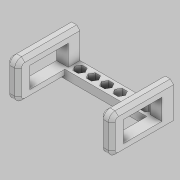
# Autodesk Inventor part: Chassis_atras_V4
Saved by Autodesk Inventor 2022.2 (Build 262287010, 287A)
## iProperties
Created: 2022-06-14
Part Number: Chassis_atras_V4
Material: Genérico
Document SubType Name: Modeling
Designer: Usuario
Density: 1 g/cm^3
Appearance: Valor por defecto
Author: Usuario
Autodesk Inventor part; units mm, degrees
ref_plane "YZ Plane" through (0, 0, 0) normal (1, 0, 0) x (0, 1, 0)
ref_plane "XZ Plane" through (0, 0, 0) normal (0, 1, 0) x (-1, 0, 0)
ref_plane "XY Plane" through (0, 0, 0) normal (0, 0, 1) x (1, 0, 0)
sketch "Boceto1" plane through (0, 0, 0) normal (0, 1, 0) x (-1, 0, 0)
  line L0 (29.505, -15) -> (44.5466, 0) construction
  line L1 (33.6552, -19.1617) -> (29.505, -15) construction
  line L2 (0, 0) -> (0, 6.3504) construction
  line L3 (0, 0) -> (0, -23.2363) construction
  line L4 (0, -14.2363) -> (24.5, -14.2363)
  line L5 (31.5, -23.2363) -> (31.5, 13.7637)
  line L6 (31.5, 13.7637) -> (24.5, 13.7637)
  line L7 (24.5, 13.7637) -> (24.5, -14.2363)
  line L8 (31.5, -23.2363) -> (0, -23.2363)
  line L9 (0, -14.2363) -> (-24.5, -14.2363)
  line L10 (-31.5, -23.2363) -> (-31.5, 13.7637)
  line L11 (-31.5, 13.7637) -> (-24.5, 13.7637)
  line L12 (-24.5, 13.7637) -> (-24.5, -14.2363)
  line L13 (-31.5, -23.2363) -> (0, -23.2363)
  dimension "d70" = 7
  dimension "d71" = 37
  dimension "d86" = 31.5
  dimension "d88" = 9
  constraints: 28 end point, 4 symmetric about line, 3 horizontal, 3 vertical, 1 perpendicular, 1 point on line
  measures "d70" distance of L5.end L6.end
  measures "d71" distance of L5.start L5.end
  measures "d86" distance of L3.end L5.start
  measures "d88" distance between parallel lines of L4 L8
extrude "Extrusión1" add sketch "Boceto1" along normal blind 5
sketch "Boceto11" plane through (0, 5, 0) normal (0, 1, 0) x (1, 0, 0)
  line L0 (-31.5, -13.7637) -> (-24.5, -13.7637) projected
  line L1 (31.5, 23.2363) -> (-31.5, 23.2363) projected
  line L2 (-31.5, -13.7637) -> (-24.5, -13.7637)
  line L3 (-24.5, -13.7637) -> (-24.5, 23.2363)
  line L4 (-24.5, 23.2363) -> (-31.5, 23.2363)
  line L5 (-31.5, 23.2363) -> (-31.5, -13.7637)
  line L6 (0, 0) -> (0, -8.2135) construction
  line L7 (31.5, -13.7637) -> (24.5, -13.7637)
  line L8 (24.5, -13.7637) -> (24.5, 23.2363)
  line L9 (24.5, 23.2363) -> (31.5, 23.2363)
  line L10 (31.5, 23.2363) -> (31.5, -13.7637)
  point P0 (31.5, 23.2363)
  point P1 (24.5, 23.2363)
  constraints: 18 end point, 6 symmetric about line, 2 parallel, 1 horizontal, 1 perpendicular, 1 point on line, 1 vertical
extrude "Extrusión7" add sketch "Boceto11" along normal blind 17.5
sketch "Boceto12" plane through (31.5, 0, 13.7637) normal (1, 0, 0) x (0, 0, -1)
  line L0 (7, 17.5) -> (30, 17.5)
  line L1 (30, 17.5) -> (30, 5)
  line L2 (30, 5) -> (7, 5)
  line L3 (7, 5) -> (7, 17.5)
  line L4 (37, 22.5) -> (0, 22.5) projected
  line L5 (18.5, 22.5) -> (18.5, 29.9213) construction
  line L6 (0, 0) -> (0, 22.5) projected
  line L7 (0, 11.25) -> (-3.0724, 11.25) construction
  point P0 (13.7637, 0)
  dimension "d74" = 12.5
  dimension "d75" = 23
  constraints: 12 end point, 2 horizontal, 2 midpoint, 2 parallel, 2 symmetric about line, 1 perpendicular, 1 vertical
  measures "d74" distance of L0.end L1.end
  measures "d75" distance of L1.end L2.end
extrude "Extrusión8" cut sketch "Boceto12" against normal through all
fillet "Empalme5" radius 4 4 edges at (-28, 0, 13.7637) (-28, 22.5, 13.7637) (28, 0, 13.7637) (28, 22.5, 13.7637)
chamfer "Chaflán3" distance 2 angle 45 20 edges at (31.5, 22.5, -6.7363) (31.5, 21.3284, 12.5921) (31.5, 11.25, 13.7637) (31.5, 1.1716, 12.5921) (31.5, 0, -6.7363) (-31.5, 22.5, -6.7363) (-31.5, 21.3284, 12.5921) (-31.5, 11.25, 13.7637) (-31.5, 1.1716, 12.5921) (-31.5, 0, -6.7363) (-24.5, 22.5, -6.7363) (-24.5, 21.3284, 12.5921) (-24.5, 11.25, 13.7637) (-24.5, 1.1716, 12.5921) (-24.5, 0, -2.2363) (24.5, 22.5, -6.7363) (24.5, 21.3284, 12.5921) (24.5, 11.25, 13.7637) (24.5, 1.1716, 12.5921) (24.5, 0, -2.2363)
sketch "Boceto13" plane through (0, 5, 0) normal (0, 1, 0) x (1, 0, 0)
  line L0 (0, 0) -> (0, -6.0566) construction
  line L1 (-2.4123, 15.9863) -> (-5.5877, 15.9863)
  line L2 (-5.5877, 15.9863) -> (-7.1754, 18.7363)
  line L3 (-7.1754, 18.7363) -> (-5.5877, 21.4863)
  line L4 (-5.5877, 21.4863) -> (-2.4123, 21.4863)
  line L5 (-2.4123, 21.4863) -> (-0.8246, 18.7363)
  line L6 (-0.8246, 18.7363) -> (-2.4123, 15.9863)
  line L7 (24.5, 23.2363) -> (-24.5, 23.2363) projected
  line L8 (-13.5877, 21.4863) -> (-10.4123, 21.4863)
  line L9 (-15.1754, 18.7363) -> (-13.5877, 21.4863)
  line L10 (-13.5877, 15.9863) -> (-15.1754, 18.7363)
  line L11 (-10.4123, 15.9863) -> (-13.5877, 15.9863)
  line L12 (-8.8246, 18.7363) -> (-10.4123, 15.9863)
  line L13 (-10.4123, 21.4863) -> (-8.8246, 18.7363)
  line L14 (-21.5877, 21.4863) -> (-18.4123, 21.4863)
  line L15 (-23.1754, 18.7363) -> (-21.5877, 21.4863)
  line L16 (-21.5877, 15.9863) -> (-23.1754, 18.7363)
  line L17 (-18.4123, 15.9863) -> (-21.5877, 15.9863)
  line L18 (-16.8246, 18.7363) -> (-18.4123, 15.9863)
  line L19 (-18.4123, 21.4863) -> (-16.8246, 18.7363)
  line L20 (2.4123, 15.9863) -> (5.5877, 15.9863)
  line L21 (5.5877, 15.9863) -> (7.1754, 18.7363)
  line L22 (7.1754, 18.7363) -> (5.5877, 21.4863)
  line L23 (5.5877, 21.4863) -> (2.4123, 21.4863)
  line L24 (2.4123, 21.4863) -> (0.8246, 18.7363)
  line L25 (0.8246, 18.7363) -> (2.4123, 15.9863)
  line L26 (13.5877, 21.4863) -> (10.4123, 21.4863)
  line L27 (15.1754, 18.7363) -> (13.5877, 21.4863)
  line L28 (13.5877, 15.9863) -> (15.1754, 18.7363)
  line L29 (10.4123, 15.9863) -> (13.5877, 15.9863)
  line L30 (8.8246, 18.7363) -> (10.4123, 15.9863)
  line L31 (10.4123, 21.4863) -> (8.8246, 18.7363)
  line L32 (21.5877, 21.4863) -> (18.4123, 21.4863)
  line L33 (23.1754, 18.7363) -> (21.5877, 21.4863)
  line L34 (21.5877, 15.9863) -> (23.1754, 18.7363)
  line L35 (18.4123, 15.9863) -> (21.5877, 15.9863)
  line L36 (16.8246, 18.7363) -> (18.4123, 15.9863)
  line L37 (18.4123, 21.4863) -> (16.8246, 18.7363)
  point P0 (-4, 18.7363)
  dimension "d87" = 5.5
  dimension "d89" = 4.5
  dimension "d90" = 4
  dimension "d93" = 8
  constraints: 74 end point, 18 symmetric about line, 2 horizontal, 1 vertical, 37 other
  measures "d87" distance between parallel lines of L4 L1
  measures "d89" distance from line of L7 point (-4, 18.736)
  measures "d90" horizontal distance of L0.start point (-4, 18.736)
  measures "d93" distance of L3.end L8.start
extrude "Extrusión9" cut sketch "Boceto13" against normal up to surface (5 mm away)
